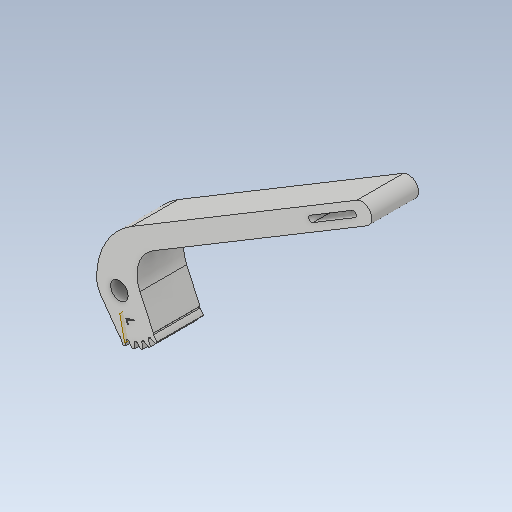
# Autodesk Inventor part: GripperLever_v2
Saved by Autodesk Inventor 2021.4 (Build 254397000, 397)
## iProperties
Created: 2022-04-22
Part Number: GripperLever_v2
Material: Generisch
Document SubType Name: Modeling
Designer: ALEX
Density: 1 g/cm^3
Appearance: Vorgabe
Mass: 2.12674 g
Surface Area: 20.0377 cm^2
Volume: 2.12674 cm^3
Di: 13,833 mm
GearThickness: 9,000 mm
Lever_Do: 8,000 mm
d: 15,000 mm
Author: ALEX
Autodesk Inventor part; units mm, degrees
ref_plane "YZ Plane" through (0, 0, 0) normal (1, 0, 0) x (0, 1, 0)
ref_plane "XZ Plane" through (0, 0, 0) normal (0, 1, 0) x (-1, 0, 0)
ref_plane "XY Plane" through (0, 0, 0) normal (0, 0, 1) x (1, 0, 0)
sketch "Skizze1" plane through (0, 0, 0) normal (0, 0, 1) x (1, 0, 0)
  circle A0 centre (0, 0) radius 6.9167 construction
  circle A1 centre (0, 0) radius 8 construction
  arc A2 (0.254, -7.0637) -> (0.067, -6.9163) centre (0.0688, -7.1063) ccw
  arc A3 (0.254, -7.0637) -> (0.662, -7.9726) centre (2.7536, -6.4875) ccw
  line L0 (0, 0) -> (1.6633, -7.8252) construction
  line L1 (0, 0) -> (0, -8) construction
  arc A4 (0.662, -7.9726) -> (1.01, -7.936) centre (0, 0) ccw
  arc A5 (1.01, -7.936) -> (1.2202, -6.9621) centre (-1.3446, -6.9182) ccw
  arc A6 (1.3724, -6.7791) -> (1.2202, -6.9621) centre (1.4102, -6.9654) ccw
  arc A7 (1.3724, -6.7791) -> (1.4381, -6.7655) centre (0, 0) ccw
  line L2 (0, 0) -> (0.8362, -7.9562) construction
  circle A8 centre (0, 0) radius 7.5 construction
  circle A9 centre (0, 0) radius 4
  circle A10 centre (0, 0) radius 1.55
  circle A11 centre (0, 0) radius 7.0477 construction
  line L3 (0.3923, -7.4897) -> (2.7536, -6.4875) construction
  arc A12 (0, -6.9167) -> (0.067, -6.9163) centre (0, 0) ccw
  line L4 (1.1734, -7.4076) -> (-1.3446, -6.9182) construction
  arc A13 (1.7171, -6.8565) -> (1.5035, -6.7513) centre (1.5448, -6.9367) ccw
  arc A14 (1.7171, -6.8565) -> (2.3052, -7.6607) centre (4.0423, -5.7732) ccw
  arc A15 (2.7519, -6.3456) -> (2.8133, -6.3187) centre (0, 0) ccw
  arc A16 (2.7519, -6.3456) -> (2.641, -6.5563) centre (2.8275, -6.52) ccw
  arc A17 (2.6379, -7.5526) -> (2.641, -6.5563) centre (0.1232, -7.0466) ccw
  arc A18 (2.3052, -7.6607) -> (2.6379, -7.5526) centre (0, 0) ccw
  arc A19 (1.4381, -6.7655) -> (1.5035, -6.7513) centre (0, 0) ccw
  arc A20 (3.1051, -6.3497) -> (2.8743, -6.2911) centre (2.9533, -6.464) ccw
  arc A21 (3.1051, -6.3497) -> (3.8475, -7.014) centre (5.1542, -4.8066) ccw
  arc A22 (4.0111, -5.6348) -> (4.0655, -5.5957) centre (0, 0) ccw
  arc A23 (4.0111, -5.6348) -> (3.9464, -5.8639) centre (4.1213, -5.7896) ccw
  arc A24 (4.1505, -6.8391) -> (3.9464, -5.8639) centre (1.5856, -6.867) ccw
  arc A25 (3.8475, -7.014) -> (4.1505, -6.8391) centre (0, 0) ccw
  arc A26 (2.8133, -6.3187) -> (2.8743, -6.2911) centre (0, 0) ccw
  arc A27 (4.3574, -5.5653) -> (4.1195, -5.5561) centre (4.2327, -5.7087) ccw
  arc A28 (4.3574, -5.5653) -> (5.2218, -6.0608) centre (6.041, -3.63) ccw
  arc A29 (5.095, -4.6777) -> (5.1401, -4.6282) centre (0, 0) ccw
  arc A30 (5.095, -4.6777) -> (5.0794, -4.9153) centre (5.235, -4.8062) ccw
  arc A31 (5.4818, -5.8267) -> (5.0794, -4.9153) centre (2.9786, -6.3873) ccw
  arc A32 (5.2218, -6.0608) -> (5.4818, -5.8267) centre (0, 0) ccw
  arc A33 (4.0655, -5.5957) -> (4.1195, -5.5561) centre (0, 0) ccw
  arc A34 (5.4193, -4.5378) -> (5.1847, -4.5781) centre (5.3271, -4.7039) ccw
  arc A35 (5.4193, -4.5378) -> (6.3678, -4.8427) centre (6.6637, -2.2947) ccw
  arc A36 (5.9562, -3.5162) -> (5.99, -3.4583) centre (0, 0) ccw
  arc A37 (5.9562, -3.5162) -> (5.9903, -3.7518) centre (6.1198, -3.6128) ccw
  arc A38 (6.5734, -4.5596) -> (5.9903, -3.7518) centre (4.2415, -5.6284) ccw
  arc A39 (6.3678, -4.8427) -> (6.5734, -4.5596) centre (0, 0) ccw
  arc A40 (5.1401, -4.6282) -> (5.1847, -4.5781) centre (0, 0) ccw
  line L5 (0, -6.9167) -> (-3.2633, -2.3133)
  line L6 (5.99, -3.4583) -> (3.635, 1.6694)
  point P0 (3.2539, -7.3084)
  point P1 (1.941, -7.2445)
  point P2 (2.6879, -7.0018)
  point P3 (2.4721, -7.6085)
  point P4 (1.6633, -7.8252)
  point P5 (4.7023, -6.4721)
  point P6 (3.4048, -6.6826)
  point P7 (4.0849, -6.2899)
  point P8 (4, -6.9282)
  point P9 (3.2539, -7.3084)
  point P10 (5.9452, -5.353)
  point P11 (4.7198, -5.8287)
  point P12 (5.3034, -5.3032)
  point P13 (5.353, -5.9452)
  point P14 (4.7023, -6.4721)
  point P15 (6.9282, -4)
  point P16 (5.8285, -4.72)
  point P17 (6.2901, -4.0846)
  point P18 (6.4721, -4.7023)
  point P19 (5.9452, -5.353)
  point P20 (0, -6.9167)
  point P21 (1.4381, -6.7655)
  point P22 (2.8133, -6.3187)
  point P23 (4.0655, -5.5957)
  point P24 (5.1401, -4.6282)
  point P25 (5.99, -3.4583)
  dimension "d0" = 13.8333
  dimension "d1" = 16
  dimension "d2" = 0.19
  dimension "d5" = 12
  dimension "d6" = 6
  dimension "d9" = 15
  dimension "d10" = 0.7854
  dimension "Lever_Do" = 8
  dimension "d17" = 3.1
  dimension "d26" = 14.0954
  dimension "beta_circ" = 48
  constraints: 94 point on circle, 41 centre point, 14 end point, 10 coincident, 9 tangent, 2 concentric, 2 equal radius, 2 point on line, 1 vertical, 108 other
  measures "d0" diameter of A0
  measures "d1" diameter of A1
  measures "d2" radius of A2
  measures "d5" angle of L0 L1
  measures "d6" angle of L1 L2
  measures "d9" diameter of A8
  measures "d10" distance of L4.start L3.start
  measures "Lever_Do" diameter of A9
  measures "d17" diameter of A10
  measures "d26" diameter of A11
extrude "Extrusion1" add sketch "Skizze1" along normal blind 9
sketch "Skizze2" plane through (0, 0, 9) normal (0, 0, 1) x (1, 0, 0)
  line L0 (0, 0) -> (44.1923, 0) construction
  arc A0 (3.635, 1.6694) -> (-3.2633, -2.3133) centre (0, 0) ccw projected
  line L1 (43.291, 35.5783) -> (45.0937, 32.5782)
  line L2 (44.4241, 33.6925) -> (1.5657, 7.9406) construction
  line L3 (0, 0) -> (0.7738, 3.9244) construction
  line L4 (44.1923, 0) -> (44.1923, 34.0782) construction
  circle A1 centre (0, 0) radius 4 construction
  line L5 (5.91, 9.0342) -> (45.0937, 32.5782)
  line L6 (43.291, 35.5783) -> (2.1398, 10.8521)
  arc A2 (2.1398, 10.8521) -> (-4, 0) centre (8.6605, 0) ccw
  arc A3 (5.91, 9.0342) -> (3.635, 1.6694) centre (8.8861, 4.0811) ccw
  circle A4 centre (0, 0) radius 1.55 construction
  line L7 (0, 0) -> (44.1923, 26.5534) construction
  dimension "d39" = 31
  dimension "d70" = 8
  dimension "d72" = 50
  dimension "d86" = 6
  dimension "d87" = 1.3
  dimension "d88" = 3.5
  constraints: 16 end point, 6 point on circle, 5 point on line, 4 tangent, 3 centre point, 3 parallel, 2 coincident, 1 horizontal, 1 midpoint, 1 perpendicular, 1 vertical
  measures "d39" angle of L0 L2
  measures "d70" diameter of A1
  measures "d72" distance of L2.start L2.end
  measures "d86" distance between parallel lines of L2 L7
  measures "d87" distance between parallel lines of L5 L2
  measures "d88" distance between parallel lines of L5 L6
extrude "Extrusion2" add sketch "Skizze2" against normal up to surface (9 mm away)
ref_plane "AdjustPlane_left" through (1.4381, -6.7655, 9) normal (0.9781476, 0.2079117, 0) x (0, 0, -1)
sketch "Sketch4" plane through (0, 0, 9) normal (0, 0, 1) x (1, 0, 0)
  line L0 (2.5, -3) -> (2.8762, -4.0337) construction
  line L1 (2.8762, -4.0337) -> (1.3727, -4.5809) construction
  line L2 (1.3727, -4.5809) -> (0.9965, -3.5472) construction
  line L3 (0.9965, -3.5472) -> (2.5, -3) construction
  line L4 (0, 0) -> (0, -3) construction
  line L5 (0, -3) -> (2.5, -3) construction
  line L6 (1.4397, -4.4725) -> (1.1424, -3.6558)
  line L7 (1.1424, -3.6558) -> (2.552, -3.1428)
  line L8 (2.552, -3.1428) -> (2.6202, -3.3301)
  line L9 (2.6202, -3.3301) -> (1.3774, -3.7824)
  line L10 (1.3774, -3.7824) -> (1.6065, -4.4118)
  line L11 (1.6065, -4.4118) -> (1.4397, -4.4725)
  dimension "d75" = 3
  dimension "d76" = 2.5
  dimension "d77" = 1.6
  dimension "d78" = 1.1
  dimension "d81" = 20
  constraints: 4 end point, 1 horizontal, 1 vertical, 2 other
  measures "d75" vertical distance of L4.start L0.start
  measures "d76" horizontal distance of L4.start L0.start
  measures "d77" distance of L0.end L1.end
  measures "d78" distance of L1.end L2.end
  measures "d81" angle of L2 L4
extrude "Extrusion3" cut sketch "Sketch4" against normal blind 0.5
thicken "Thicken1" operation add thickness 0.4 both sides no extend neighbours yes toward (0, 0, -1) faces at (17.1136, 18.4882, 9)
thicken "Thicken2" operation add thickness 0.4 both sides no extend neighbours yes toward (0, 0, 1) faces at (17.1136, 18.4882, 0)
sketch "Sketch5" plane through (45.0937, 32.5782, 0.4) normal (0.5150381, -0.8571673, 0) x (0.8571673, 0.5150381, 0)
  circle A0 centre (-31.0731, 4.1) radius 2.5
  point P0 (-55.4318, -0.4)
  dimension "d89" = 5
  constraints: 2 coincident, 1 centre point, 1 other
  measures "d89" diameter of A0
extrude "Extrusion4" cut sketch "Sketch5" against normal blind 2
sketch "Sketch6" plane through (2.1398, 10.8521, 8.6) normal (0, 0, 1) x (0.8571673, 0.5150381, 0)
  line L0 (48.0083, -3.5) -> (48.0083, 0) construction
  line L1 (48.0083, -1.75) -> (33.0083, -1.75) construction
  line L2 (44.5083, -1.75) -> (35.9083, -1.75) construction
  line L3 (44.5083, -1.25) -> (35.9083, -1.25)
  line L4 (35.9083, -2.25) -> (44.5083, -2.25)
  arc A0 (44.5083, -2.25) -> (44.5083, -1.25) centre (44.5083, -1.75) ccw
  arc A1 (35.9083, -1.25) -> (35.9083, -2.25) centre (35.9083, -1.75) ccw
  point P0 (-7.4235, -8.2)
  point P1 (40.2083, -1.75)
  dimension "d92" = 15
  dimension "d93" = 1
  dimension "d94" = 8.6
  dimension "d95" = 7.8
  constraints: 10 end point, 4 point on circle, 4 tangent, 2 centre point, 2 midpoint, 2 point on line, 1 horizontal, 1 parallel
  measures "d92" distance of L1.start L1.end
  measures "d93" distance between parallel lines of L4 L3
  measures "d94" distance of L2.end L2.start
  measures "d95" distance from line of L0 point (40.208, -1.75)
extrude "Extrusion5" cut sketch "Sketch6" against normal through all
fillet "Fillet1" radius 1.75 2 edges at (43.291, 35.5783, 4.5) (45.0937, 32.5782, 4.5)
equation "\"d9\" = d"
equation "\"Gear_r\" = 0.38"
equation "\"Gear_R\" = 5.1303"
equation "\"modul\" = 0.5"
equation "\"Sp\" = 1.57008"
equation "\"TotalAngle\" = 48deg"
equation "\"alpha\" = 12deg"
equation "\"Do\" = 16"
equation "\"Di\" = 13.83333"
equation "\"p\" = 1.570796"
equation "\"delta_f\" = 0.19"
equation "\"Db\" = 14.09539"
equation "\"Kopfspiel\" = 0.58333"
equation "\"beta_circ_max\" = 60deg"
equation "\"d\" = 15"
